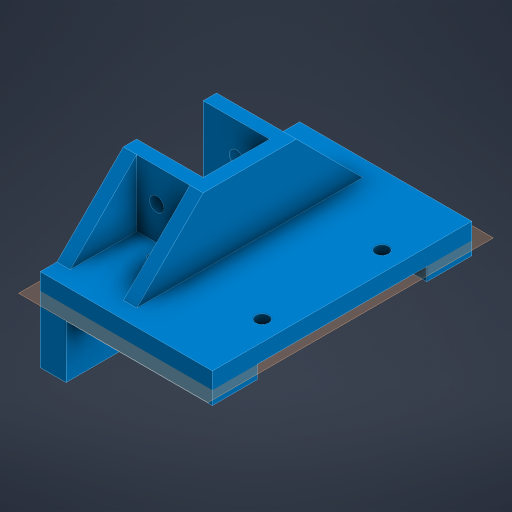
# Autodesk Inventor part: XY Rail Bracket
Saved by Autodesk Inventor 2024.2 (Build 282272000, 272)
## iProperties
Created: 2024-10-06
Part Number: XY Rail Bracket
Material: Generic
Document SubType Name: Modeling
Designer: jerem
Density: 1 g/cm^3
Appearance: Default
Author: jerem
Autodesk Inventor part; units mm, degrees
ref_plane "YZ Plane" through (0, 0, 0) normal (1, 0, 0) x (0, 1, 0)
ref_plane "XY Plane" through (0, 0, 0) normal (0, 0, 1) x (1, 0, 0)
sketch "Sketch1" plane through (0, 0, 0) normal (0, 1, 0) x (-1, 0, 0)
  line L0 (16, 18) -> (16, -18) construction
  circle A0 centre (16, -18) radius 2
  line L1 (16, 0) -> (0, 0) construction
  line L2 (-16, 0) -> (0, 0) construction
  line L3 (-16, 18) -> (-16, -18) construction
  circle A1 centre (-16, 18) radius 2
  circle A2 centre (-16, -18) radius 2
  line L4 (22, -25.5) -> (-22, -25.5) construction
  line L5 (-22, -25.5) -> (22, -25.5)
  line L6 (-22, -25.5) -> (-22, 25.5)
  line L7 (22, -25.5) -> (-22, 25.5) construction
  line L8 (-22, -25.5) -> (22, 25.5) construction
  circle A3 centre (16, 18) radius 2
  line L9 (-22, 25.5) -> (22, 25.5) construction
  line L10 (-22, 25.5) -> (22, 25.5)
  circle A4 centre (16, -18) radius 4
  circle A5 centre (-16, -18) radius 4
  circle A6 centre (-16, 18) radius 4
  circle A7 centre (16, 18) radius 4
  line L11 (22, -25.5) -> (-22, -25.5)
  line L12 (-22, -25.5) -> (-22, -39)
  line L13 (-22, -39) -> (22, -39)
  line L14 (22, -39) -> (22, -25.5)
  line L15 (22, 25.5) -> (-22, 25.5)
  line L16 (-22, 25.5) -> (-22, 39)
  line L17 (-22, 39) -> (22, 39)
  line L18 (22, 39) -> (22, 25.5)
  line L19 (22, 0) -> (9.75, 0) construction
  line L20 (9.75, 0) -> (9.75, 10) construction
  line L21 (9.75, 0) -> (9.75, -10) construction
  line L22 (29.75, 10) -> (9.75, 10)
  line L23 (9.75, 10) -> (9.75, 14)
  line L24 (9.75, 14) -> (29.75, 14)
  line L25 (9.75, -10) -> (29.75, -10)
  line L26 (9.75, -10) -> (9.75, -14)
  line L27 (9.75, -14) -> (29.75, -14)
  line L28 (9.75, 10) -> (5.75, 10)
  line L29 (5.75, 10) -> (5.75, -10)
  line L30 (5.75, -10) -> (9.75, -10)
  line L31 (9.75, -10) -> (9.75, 10)
  line L32 (9.75, 14) -> (5.75, 14)
  line L33 (5.75, 14) -> (5.75, 10)
  line L34 (5.75, -10) -> (5.75, -14)
  line L35 (5.75, -14) -> (9.75, -14)
  line L36 (22, 0) -> (16, 0) construction
  line L37 (34.75, 46.236) -> (34.75, -49.0008) construction
  line L38 (22, 39) -> (29.75, 39)
  line L39 (29.75, 39) -> (29.75, -39)
  line L40 (29.75, -39) -> (22, -39)
  line L41 (22, 25.5) -> (22, -25.5)
  point P0 (9.75, -10)
  point P1 (9.75, 0)
  dimension "d0" = 36
  dimension "d1" = 4
  dimension "d2" = 4
  dimension "d3" = 36
  dimension "d4" = 4
  dimension "d5" = 4
  dimension "d6" = 32
  dimension "d7" = 51
  dimension "d8" = 44
  dimension "d9" = 2
  dimension "d10" = 2
  dimension "d11" = 2
  dimension "d12" = 2
  dimension "d13" = 13.5
  dimension "d14" = 13.5
  dimension "d19" = 4
  dimension "d20" = 20
  dimension "d75" = 9.75
  dimension "d79" = 20
  dimension "d80" = 34.75
  constraints: 84 end point, 14 perpendicular, 12 point on line, 11 horizontal, 9 equal length, 8 centre point, 6 midpoint, 4 vertical, 3 collinear, 2 coincident, 2 tangent
  measures "d0" distance of L3.start L3.end
  measures "d1" diameter of A1
  measures "d2" diameter of A2
  measures "d3" distance of L0.start L0.end
  measures "d4" diameter of A3
  measures "d5" diameter of A0
  measures "d6" distance between parallel lines of L0 L3
  measures "d7" distance between parallel lines of L4 L9
  measures "d8" distance of L7.start L8.start
  measures "d9" radial gap between concentric circles of A4 A0
  measures "d10" radial gap between concentric circles of A5 A2
  measures "d11" radial gap between concentric circles of A6 A1
  measures "d12" radial gap between concentric circles of A3 A7
  measures "d13" distance between parallel lines of L4 L13
  measures "d14" distance between parallel lines of L9 L17
  measures "d19" distance of L30.end L29.end
  measures "d20" distance of L29.end L28.end
  measures "d75" distance from line of point (0, 0) L20
  measures "d79" distance between parallel lines of L20 L39
  measures "d80" distance from line of point (0, 0) L37
extrude "Extrusion1" add sketch "Sketch1" against normal blind 4 contours L5 L14 L13 L12 | L16 L17 L18 L10
extrude "Extrusion2" add sketch "Sketch1" along normal blind 5 contours A0 | A1 | A2 | A4 | A7 | L6 L10 L41 L24 L32 L33 L29 L34 L35 L27 L5 | L5 L14 L13 L12 | L41 L27 L39 L40 L14 | L16 L17 L18 L10 | L41 L25 L39 L27 | L27 L26 L25 L41 | L18 L38 L39 L24 L41 | L41 L22 L39 L25 | L25 L31 L22 L41 | L41 L22 L23 L24 | L24 L39 L22 L41 | L35 L34 L30 L26 | L30 L29 L28 L31 | L28 L33 L32 L23 | A3 | A5 | A6
extrude "Extrusion14" add sketch "Sketch1" against normal blind 20 contours L41 L27 L39 L40 L14 | L41 L25 L39 L27 | L18 L38 L39 L24 L41 | L41 L22 L39 L25 | L24 L39 L22 L41
extrude "Extrusion3" add sketch "Sketch1" along normal blind 20 from surface at 5 contours L41 L25 L39 L27 | L27 L26 L25 L41 | L41 L22 L23 L24 | L24 L39 L22 L41 | L35 L34 L30 L26 | L30 L29 L28 L31 | L28 L33 L32 L23
extrude "Extrusion4" cut sketch "Sketch1" along normal through all contours A0 | A1 | A2 | A3
sketch "Sketch3" plane through (-9.75, 5, 10) normal (0, 0, -1) x (-1, 0, 0)
  circle A0 centre (10, 10) radius 2.2
  circle A1 centre (10, 10) radius 4.2
  line L0 (20, 0) -> (20, 20) projected
  line L1 (0, 0) -> (20, 0) projected
  dimension "d63" = 4.4
  dimension "d64" = 2
  dimension "d94" = 10
  dimension "d101" = 10
  constraints: 2 centre point, 1 coincident
  measures "d63" diameter of A0
  measures "d64" radial gap between concentric circles of A1 A0
  measures "d94" distance from line of L0 A0.centre
  measures "d101" distance from line of L1 A0.centre
sketch "Sketch4" plane through (-29.75, -20, -39) normal (-1, 0, 0) x (0, 0, 1)
  line L0 (53, 45) -> (72.9998, 25.0002)
  line L1 (53, 45) -> (81.284, 45) construction
  line L2 (72.9998, 25.0002) -> (53, 25.0002)
  line L3 (53, 25.0002) -> (53, 45)
  point P0 (39, 20)
  dimension "d95" = 28.284
  dimension "d96" = 45
  constraints: 8 end point, 2 horizontal, 1 equal length, 1 vertical
  measures "d95" distance of L0.start L0.end
  measures "d96" angle of L0 L1
extrude "Extrusion15" cut sketch "Sketch3" against normal through all contours A0
extrude "Extrusion16" add sketch "Sketch4" against normal blind 4
extrude "Extrusion17" add sketch "Sketch4" along normal blind 4 from surface at -24
mirror "Mirror1" about plane through (0, 0, 0) normal (0, 0, 1) of "Extrusion16", "Extrusion17", "Extrusion15"
equation "\"d2\" = d1"
equation "\"d4\" = d1"
equation "\"d5\" = d1"
equation "\"d10\" = d9"
equation "\"d11\" = d9"
equation "\"d12\" = d9"
equation "\"d14\" = d13"
body "Solid1"
